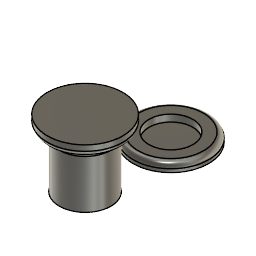
Rotary Engrave Coin Holder Parameterized (Autodesk Fusion 360 design; units mm, degrees)
Autodesk Fusion 360 part; units mm, degrees
sketch "Sketch1" plane through (0, 0, 0) normal (0, 0, 1) x (1, 0, 0)
  circle A0 centre (0, 0) radius 15
  dimension "d10" = 30
  constraint coincident A0.centre origin
  measures "d10" diameter of A0
extrude "Extrude1" add sketch "Sketch1" along normal blind 30 makes body 1
ref_plane "WorkPlane1" through (0, 0, 34.0415) normal (0, 0, 1) x (1, 0, 0)
sketch "Sketch2" plane through (0, 0, 34.0415) normal (0, 0, 1) x (1, 0, 0)
  circle A0 centre (0, 0) radius 22
  dimension "d16" = 44
  constraint coincident A0.centre origin
  measures "d16" diameter of A0
extrude "Extrude2" add sketch "Sketch2" along normal blind 5 separate body makes body 2
loft "Loft1" add section 1 face at (3.6653, 3.4009, 30) section 2 face at (5.8152, -3.0625, 34.0415) on bodies 1 2 bodies 1 2
sketch "Sketch3" plane through (0, 0, 39.0415) normal (0, 0, 1) x (-1, 0, 0)
  circle A0 centre (0, 0) radius 22
  circle A1 centre (0, 0) radius 12.775
  dimension "d19" = 25.55
  constraint coincident A0.centre A1.centre
  measures "d19" diameter of A1
extrude "Extrude3" cut sketch "Sketch3" against normal up to surface (38.0415 mm away) from surface at -1 contours A1 bodies 1
sketch "Sketch5" plane through (0, 0, 0) normal (0, 0, 1) x (1, 0, 0)
  circle A0 centre (0, 50) radius 22
  dimension "d26" = 44
  measures "d26" diameter of A0
extrude "Extrude5" add sketch "Sketch5" along normal blind 5 separate body makes body 3
sketch "Sketch7" plane through (0, 0, 0) normal (0, 0, -1) x (1, 0, 0)
  circle A0 centre (0, -50) radius 22
  circle A1 centre (0, -50) radius 12.775
  dimension "d39" = 25.55
  measures "d39" diameter of A1
extrude "Extrude7" cut sketch "Sketch7" against normal blind 5 from surface at -1 contours A1 bodies 3
fillet "Fillet1" radius 3 1 edges at (-20.5112, -7.9555, 34.0415) on bodies 1
fillet "Fillet2" radius 3 1 edges at (-13.9849, -5.4242, 30) on bodies 1
fillet "Fillet3" radius 3 1 edges at (-20.5112, 42.0445, 5) on bodies 3
equation "DiameterBase = 30 mm"
equation "DiameterCoin = 44 mm"
equation "DiameterMagnet = 25.55 mm"
equation "HeightMagnet = 3.2 mm"
equation "HeightBase = 30 mm"
equation "HeightJigPlate = 5 mm"
equation "d10 = DiameterBase"
equation "d11 = HeightBase"
equation "AngleLoft = 30 deg"
equation "HeightOffset = abs(DiameterBase - DiameterCoin) / 2 * tan(AngleLoft)"
equation "d15 = HeightOffset"
equation "d16 = DiameterCoin"
equation "d17 = HeightJigPlate"
equation "d19 = DiameterMagnet"
equation "d26 = DiameterCoin"
equation "d27 = HeightJigPlate"
equation "FilletSize = 3 mm"
equation "d34 = FilletSize"
equation "d36 = FilletSize"
equation "d38 = FilletSize"
equation "d39 = DiameterMagnet"
equation "d41 = -HeightJigPlate"
